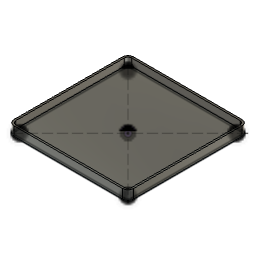
skvrampel-tray-v1 (Autodesk Fusion 360 design; units mm, degrees)
part number: 2025-05-31-23-56-43-537
Autodesk Fusion 360 part; units mm, degrees
sketch "Bottom and Walls" plane through (0, 0, 0) normal (0, 0, 1) x (1, 0, 0)
  line L0 (59, 65) -> (-59, 65)
  line L1 (-65, 59) -> (-65, -59)
  line L2 (-59, -65) -> (59, -65)
  line L3 (65, -59) -> (65, 59)
  line L4 (65, 65) -> (-65, -65) construction
  line L5 (-65, 65) -> (65, -65) construction
  arc A0 (-59, 65) -> (-65, 59) centre (-59, 59) ccw
  arc A1 (65, 59) -> (59, 65) centre (59, 59) ccw
  arc A2 (59, -65) -> (65, -59) centre (59, -59) ccw
  arc A3 (-65, -59) -> (-59, -65) centre (-59, -59) ccw
  line L6 (-63, 59) -> (-63, -59)
  arc A4 (-63, -59) -> (-59, -63) centre (-59, -59) ccw
  line L7 (-59, -63) -> (59, -63)
  arc A5 (59, -63) -> (63, -59) centre (59, -59) ccw
  line L8 (63, -59) -> (63, 59)
  arc A6 (63, 59) -> (59, 63) centre (59, 59) ccw
  line L9 (59, 63) -> (-59, 63)
  arc A7 (-59, 63) -> (-63, 59) centre (-59, 59) ccw
  dimension "d6" = 130
  dimension "d7" = 130
  dimension "d8" = 6
  dimension "d9" = -2
  constraint horizontal L0
  constraint perpendicular L0 L1
  constraint parallel L0 L2
  constraint parallel L1 L3
  constraint coincident L4 origin
  constraint coincident L5 origin
  constraint coincident L5.start L1
  constraint coincident L5.start L0
  constraint tangent L1 A0
  constraint tangent L0 A0
  constraint coincident L4.start L3
  constraint coincident L4.start L0
  constraint tangent L3 A1
  constraint tangent L0 A1
  constraint equal A0 A1
  constraint coincident L5.end L3
  constraint coincident L5.end L2
  constraint tangent L3 A2
  constraint tangent L2 A2
  constraint equal A0 A2
  constraint coincident L4.end L2
  constraint coincident L4.end L1
  constraint tangent L2 A3
  constraint tangent L1 A3
  constraint equal A0 A3
  measures "d6" distance of L4.end L5.end
  measures "d7" distance of L5.start L4.end
  measures "d8" radius of A0
extrude "Extrude2" add sketch "Bottom and Walls" along normal blind 10 makes body 1
extrude "Extrude3" add sketch "Bottom and Walls" along normal blind 2 contours L6 A4 L7 A5 L8 A6 L9 A7 bodies 1
extrude "Extrude4" add sketch "Bottom and Walls" along normal blind 2 separate body contours L6 A4 L7 A5 L8 A6 L9 A7 makes body 2
named bodies: "Walls", "Bottom"
